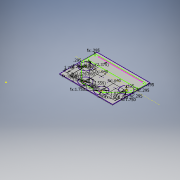
# Autodesk Inventor part: track side panel V2
Saved by Autodesk Inventor 2016 (Build 200138000, 138)
## iProperties
Created: 2015-10-10
Part Number: track side panel V2
Material: Generic
Document SubType Name: Modeling
Designer: Delta
Density: 1 g/cm^3
Appearance: Default
Author: Delta
Autodesk Inventor part; units mm, degrees
ref_plane "YZ Plane" through (0, 0, 0) normal (1, 0, 0) x (0, 1, 0)
ref_plane "XZ Plane" through (0, 0, 0) normal (0, 1, 0) x (-1, 0, 0)
ref_plane "XY Plane" through (0, 0, 0) normal (0, 0, 1) x (1, 0, 0)
sketch "Sketch1" plane through (0, 0, 0) normal (0, 1, 0) x (-1, 0, 0)
  line L0 (-77.6185, -139.5068) -> (-293.5185, -139.5068)
  line L1 (-293.5185, -139.5068) -> (-293.5185, -291.9068)
  line L2 (-293.5185, -291.9068) -> (-77.6185, -291.9068)
  line L3 (-77.6185, -291.9068) -> (-77.6185, -139.5068)
  point P0 (0, 0)
  dimension "d0" = 215.9
  dimension "d1" = 152.4
  constraints: 8 end point, 2 parallel, 1 horizontal, 1 perpendicular
  measures "d0" distance of L2.end L1.end
  measures "d1" distance of L1.end L0.end
extrude "Extrusion1" add sketch "Sketch1" along normal blind 3.175
sketch "Sketch2" plane through (0, 3.175, 0) normal (0, 1, 0) x (1, 0, 0)
  line L0 (77.6185, 291.9068) -> (77.6185, 139.5068) projected
  line L1 (77.6185, 139.5068) -> (293.5185, 139.5068) projected
  line L2 (293.5185, 139.5068) -> (293.5185, 291.9068) projected
  line L3 (293.5185, 291.9068) -> (77.6185, 291.9068) projected
  point P0 (0, 0)
  point P1 (156.9685, 165.5068)
  point P2 (104.9685, 218.5068)
  point P3 (269.9685, 218.5068)
  point P4 (221.9685, 165.5068)
  dimension "d4" = 144.35
  dimension "d5" = 26
  dimension "d7" = 79
  dimension "d19" = 27.35
  dimension "d20" = 79
  dimension "d21" = 26
  dimension "d22" = 79.35
  dimension "d23" = 192.35
  measures "d4" distance from line of L0 point (221.968, 165.507)
  measures "d5" distance from line of L1 point (221.968, 165.507)
  measures "d7" distance from line of L1 point (269.968, 218.507)
  measures "d19" distance from line of L0 point (104.968, 218.507)
  measures "d20" distance from line of L1 point (104.968, 218.507)
  measures "d21" distance from line of L1 point (156.968, 165.507)
  measures "d22" distance from line of L0 point (156.968, 165.507)
  measures "d23" distance from line of L0 point (269.968, 218.507)
hole "Hole1" at (156.9685, 3.175, -165.5068) at (104.9685, 3.175, -218.5068) at (269.9685, 3.175, -218.5068) at (221.9685, 3.175, -165.5068) direction (0, -1, 0) diameter 6 end through all
sketch "Sketch3" plane through (0, 3.175, 0) normal (0, 1, 0) x (1, 0, 0)
  line L0 (156.9685, 158.0068) -> (221.9685, 158.0068)
  circle A0 centre (221.9685, 165.5068) radius 3 projected
  circle A1 centre (104.3905, 218.5068) radius 3
  circle A2 centre (156.9685, 165.5068) radius 3 projected
  line L1 (151.4095, 160.4723) -> (145.8978, 166.5581)
  line L2 (227.8466, 160.8487) -> (232.9461, 167.2839)
  line L3 (77.6185, 139.5068) -> (293.5185, 139.5068)
  line L4 (293.5185, 139.5068) -> (293.5185, 291.9068)
  line L5 (293.5185, 291.9068) -> (77.6185, 291.9068)
  line L6 (77.6185, 291.9068) -> (77.6185, 139.5068)
  arc A3 (151.4095, 160.4723) -> (156.9685, 158.0068) centre (156.9685, 165.5068) ccw
  arc A4 (285.8541, 234.0487) -> (286.0149, 234.2591) centre (279.976, 238.7068) ccw
  line L7 (48.2791, 233.5068) -> (391.5458, 233.5068) construction
  arc A5 (221.9685, 158.0068) -> (227.8466, 160.8487) centre (221.9685, 165.5068) ccw
  line L8 (90.6742, 246.2068) -> (279.976, 246.2068)
  arc A6 (88.4435, 245.8674) -> (89.1827, 246.2068) centre (87.4992, 248.8988) ccw
  arc A7 (282.3943, 247.7992) -> (282.8225, 246.2068) centre (285.5693, 247.7992) ccw
  arc A8 (148.7259, 158.0419) -> (156.9685, 154.3863) centre (156.9685, 165.5068) ccw
  line L9 (156.9685, 154.3863) -> (221.9685, 154.3863)
  arc A9 (221.9685, 154.3863) -> (230.6842, 158.6001) centre (221.9685, 165.5068) ccw
  arc A10 (291.0908, 238.7068) -> (290.9416, 240.5219) centre (279.976, 238.7068) ccw
  line L10 (274.8873, 282.434) -> (98.1672, 282.434)
  line L11 (283.4416, 282.434) -> (274.8873, 282.434)
  line L12 (87.0466, 282.434) -> (98.1672, 282.434)
  circle A11 centre (269.9685, 218.5068) radius 3 projected
  line L13 (269.9685, 218.5068) -> (278.4956, 210.4264)
  line L14 (230.6842, 158.6001) -> (278.4956, 210.4264)
  line L15 (276.6668, 208.4441) -> (288.7468, 219.8795)
  line L16 (293.5185, 139.5068) -> (293.5185, 291.9068) projected
  line L17 (291.0908, 238.7068) -> (291.0908, 225.3261)
  line L18 (290.9416, 240.5219) -> (290.9416, 274.941)
  arc A12 (290.9416, 274.941) -> (283.4416, 282.434) centre (283.4486, 274.941) ccw
  line L19 (104.3905, 218.5068) -> (95.8634, 210.4264)
  line L20 (148.7259, 158.0419) -> (95.8634, 210.4264)
  line L21 (97.2189, 209.0832) -> (81.9058, 223.5361)
  line L22 (77.6185, 291.9068) -> (77.6185, 139.5068) projected
  line L23 (79.5536, 238.7068) -> (79.5536, 228.9904)
  line L24 (79.5536, 238.7068) -> (79.5536, 274.941)
  line L25 (87.0466, 282.434) -> (87.0466, 282.434)
  arc A13 (87.0466, 282.434) -> (79.5536, 274.941) centre (87.0466, 274.941) ccw
  arc A14 (288.7468, 219.8795) -> (291.0908, 225.3261) centre (283.5908, 225.3261) ccw
  arc A15 (79.5536, 228.9904) -> (81.9058, 223.5361) centre (87.0536, 228.9904) ccw
  line L26 (90.5024, 222.3303) -> (90.6742, 222.1407)
  arc A16 (79.6034, 239.7581) -> (79.5536, 238.7068) centre (90.6742, 238.7068) ccw
  line L27 (90.6742, 246.2068) -> (98.8849, 246.2068)
  line L28 (240.7374, 246.2068) -> (279.976, 246.2068)
  line L29 (271.4881, 215.9202) -> (272.0071, 216.5751)
  line L30 (285.4247, 233.5068) -> (285.8541, 234.0487)
  line L31 (85.2649, 233.5068) -> (85.1151, 233.6723)
  circle A17 centre (104.9685, 218.5068) radius 3 construction
  point P0 (0, 0)
  point P1 (79.5536, 282.434)
  dimension "d24" = 7.5
  dimension "d33" = 7.5
  dimension "d40" = 98.7582
  dimension "d72" = 6
  dimension "d90" = 3.175
  dimension "d91" = 3.175
  dimension "d93" = 7.5
  dimension "d96" = 52.578
  dimension "d98" = 11.7475
  dimension "d99" = 7.493
  dimension "d101" = 11.7475
  dimension "d102" = 7.493
  dimension "d103" = 7.5
  dimension "d104" = 7.5
  dimension "d106" = 6
  constraints: 60 end point, 31 point on circle, 14 centre point, 12 point on line, 12 tangent, 6 horizontal, 4 collinear, 3 parallel, 2 coincident, 2 vertical, 1 perpendicular, 4 other
  measures "d24" distance from line of L0 A0.centre
  measures "d33" radius of A4
  measures "d40" distance of L1.start L31.end
  measures "d72" diameter of A2
  measures "d90" radius of A6
  measures "d91" radius of A7
  measures "d93" radius of A5
  measures "d96" horizontal distance of L19.start A3.centre
  measures "d98" distance of L13.start L13.end
  measures "d99" radius of A12
  measures "d101" distance of L19.start L19.end
  measures "d102" radius of A13
  measures "d103" radius of A14
  measures "d104" radius of A15
  measures "d106" diameter of A1
extrude "Extrusion3" [suppressed]
sketch "Sketch5" plane through (0, 3.175, 0) normal (0, 1, 0) x (1, 0, 0)
  circle A0 centre (104.9685, 218.5068) radius 3 projected
  circle A1 centre (104.9685, 218.5068) radius 22.225
  circle A2 centre (156.9685, 165.5068) radius 3 projected
  circle A3 centre (156.9685, 165.5068) radius 22.225
  circle A4 centre (221.9685, 165.5068) radius 3 projected
  circle A5 centre (221.9685, 165.5068) radius 22.225
  circle A6 centre (269.9685, 218.5068) radius 3 projected
  circle A7 centre (269.9685, 218.5068) radius 22.225
  line L0 (156.9685, 158.0068) -> (221.9685, 158.0068) projected
  line L1 (274.8943, 278.8204) -> (98.1742, 278.8204) projected
  point P0 (0, 0)
  point P1 (130.9685, 202.4568)
  point P2 (243.9685, 202.4568)
  point P3 (205.7185, 215.1568)
  point P4 (189.4685, 168.1668)
  point P5 (173.2185, 215.1568)
  dimension "d45" = 44.45
  dimension "d47" = 44.45
  dimension "d48" = 44.45
  dimension "d49" = 44.45
  dimension "d50" = 57.15
  dimension "d52" = 65
  dimension "d53" = 16.25
  dimension "d54" = 16.25
  dimension "d55" = 57.15
  dimension "d56" = 44.45
  dimension "d58" = 52
  dimension "d59" = 26
  dimension "d60" = 44.45
  dimension "d61" = 26
  dimension "d62" = 32.5
  dimension "d63" = 10.16
  dimension "d95" = 60.3136
  constraints: 4 centre point, 4 coincident
  measures "d45" diameter of A1
  measures "d47" diameter of A3
  measures "d48" diameter of A5
  measures "d49" diameter of A7
  measures "d50" distance from line of L0 point (173.218, 215.157)
  measures "d52" distance of A5.centre A3.centre
  measures "d53" horizontal distance of point (173.218, 215.157) A3.centre
  measures "d54" horizontal distance of A5.centre point (205.718, 215.157)
  measures "d55" distance from line of L0 point (205.718, 215.157)
  measures "d56" distance from line of L0 point (130.968, 202.457)
  measures "d58" horizontal distance of A3.centre A1.centre
  measures "d59" horizontal distance of point (130.968, 202.457) A1.centre
  measures "d60" distance from line of L0 point (243.968, 202.457)
  measures "d61" horizontal distance of A7.centre point (243.968, 202.457)
  measures "d62" horizontal distance of A3.centre point (189.468, 168.167)
  measures "d63" distance from line of L0 point (189.468, 168.167)
  measures "d95" distance from line of A1.centre L1
hole "Hole2" at (130.9685, 3.175, -202.4568) at (243.9685, 3.175, -202.4568) at (205.7185, 3.175, -215.1568) at (189.4685, 3.175, -168.1668) at (173.2185, 3.175, -215.1568) direction (0, -1, 0) diameter 3 end through all
sketch "Sketch7" plane through (0, 3.175, 0) normal (0, 1, 0) x (1, 0, 0)
  circle A0 centre (156.9685, 165.5068) radius 3 projected
  line L0 (156.9685, 158.0068) -> (221.9685, 158.0068) projected
  circle A1 centre (156.9685, 178.0036) radius 2.9972
  line L1 (153.9713, 178.0036) -> (153.9713, 165.3773)
  line L2 (159.9657, 178.0043) -> (159.9685, 165.5075)
  circle A2 centre (221.9713, 178.0036) radius 2.9972
  circle A3 centre (221.9685, 165.5068) radius 3 projected
  line L3 (218.9741, 178.016) -> (218.9741, 165.3232)
  line L4 (224.9685, 178.0036) -> (224.9685, 165.5068)
  point P0 (0, 0)
  point P1 (218.9685, 165.5082)
  dimension "d76" = 5.9944
  dimension "d77" = 12.4968
  dimension "d78" = 5.9944
  dimension "d79" = 12.4968
  dimension "d88" = 6
  constraints: 9 point on circle, 8 end point, 3 vertical, 2 centre point, 1 tangent, 3 other
  measures "d76" diameter of A1
  measures "d77" distance of A0.centre A1.centre
  measures "d78" diameter of A2
  measures "d79" distance of A3.centre A2.centre
  measures "d88" diameter of A0
extrude "Extrusion4" cut sketch "Sketch7" against normal blind 25.4 contours A0 L1 A1 L2 | A1
sketch "Sketch8" plane through (0, 3.175, 0) normal (0, 1, 0) x (1, 0, 0)
  arc A0 (224.9685, 178.0036) -> (218.9741, 177.9913) centre (221.9713, 178.0036) ccw
  circle A1 centre (221.9685, 165.5068) radius 3
  line L0 (218.9741, 178.016) -> (218.9741, 165.3232)
  line L1 (224.9685, 178.0036) -> (224.9685, 165.5068)
  point P0 (0, 0)
  point P1 (218.9685, 165.5082)
  dimension "d82" = 5.9944
  dimension "d83" = 12.4968
  constraints: 6 point on circle, 4 end point, 2 centre point, 2 vertical, 1 point on line
  measures "d82" diameter of A0
  measures "d83" distance of A1.centre A0.centre
extrude "Extrusion5" cut sketch "Sketch8" against normal blind 25.4 contours L1 A1 L0 A0 | A1 L0 picked at (221.9464, 164.5591)
sketch "Sketch9" plane through (0, 3.175, 0) normal (0, 1, 0) x (1, 0, 0)
  point P0 (0, 0)
equation "\"d33\" = d32"
equation "\"d101\" = d98"
equation "\"d47\" = d45"
equation "\"d48\" = d45"
equation "\"d49\" = d48"
equation "\"d53\" = 0.25 * d52"
equation "\"d54\" = d53"
equation "\"d55\" = d50"
equation "\"d59\" = 0.5 * d58"
equation "\"d60\" = d56"
equation "\"d61\" = d59"
equation "\"d62\" = 0.5 * d52"
equation "\"d78\" = d76"
equation "\"d79\" = d77"
equation "\"d82\" = d84"
equation "\"d83\" = d85"
equation "\"d32\" = 7.5"
equation "\"d84\" = 5.9944"
equation "\"d85\" = 12.4968"
body "Solid1"
